Autodesk Fusion 360 part; units mm, degrees
(part 4 of 7)
  line L862 (59.3577, -70.4134) -> (59.3622, -70.4873)
  line L863 (59.3622, -70.4873) -> (59.3692, -70.5616)
  line L864 (59.3692, -70.5616) -> (59.3786, -70.6363)
  line L865 (59.3786, -70.6363) -> (59.3901, -70.7113)
  line L866 (59.3901, -70.7113) -> (59.4036, -70.7865)
  line L867 (59.4036, -70.7865) -> (59.4191, -70.8621)
  line L868 (59.4191, -70.8621) -> (59.4365, -70.9378)
  line L869 (59.4365, -70.9378) -> (59.4556, -71.0137)
  line L870 (59.4556, -71.0137) -> (59.4765, -71.0898)
  line L871 (59.4765, -71.0898) -> (59.6154, -71.1105)
  line L872 (59.6154, -71.1105) -> (59.7546, -71.1291)
  line L873 (59.7546, -71.1291) -> (59.8941, -71.1456)
  line L874 (59.8941, -71.1456) -> (59.9342, -71.0776)
  line L875 (59.9342, -71.0776) -> (59.9726, -71.0093)
  line L876 (59.9726, -71.0093) -> (60.0092, -70.9408)
  line L877 (60.0092, -70.9408) -> (60.044, -70.872)
  line L878 (60.044, -70.872) -> (60.0768, -70.8029)
  line L879 (60.0768, -70.8029) -> (60.1076, -70.7336)
  line L880 (60.1076, -70.7336) -> (60.1362, -70.6639)
  line L881 (60.1362, -70.6639) -> (60.1624, -70.5941)
  line L882 (60.1624, -70.5941) -> (60.1862, -70.524)
  line L883 (60.1862, -70.524) -> (60.207, -70.4536)
  line L884 (60.207, -70.4536) -> (60.2243, -70.3828)
  line L885 (60.2243, -70.3828) -> (60.2364, -70.3117)
  line L886 (60.2364, -70.3117) -> (60.2724, -69.8659)
  line L887 (60.2724, -69.8659) -> (60.483, -69.8801)
  line L888 (60.483, -69.8801) -> (60.694, -69.8888)
  line L889 (60.694, -69.8888) -> (60.9051, -69.8919)
  line L890 (60.9051, -69.8919) -> (61.1162, -69.8895)
  line L891 (61.1162, -69.8895) -> (61.1273, -70.3366)
  line L892 (61.1273, -70.3366) -> (61.1353, -70.4083)
  line L893 (61.1353, -70.4083) -> (61.1487, -70.4799)
  line L894 (61.1487, -70.4799) -> (61.1655, -70.5513)
  line L895 (61.1655, -70.5513) -> (61.1853, -70.6227)
  line L896 (61.1853, -70.6227) -> (61.2076, -70.6939)
  line L897 (61.2076, -70.6939) -> (61.2323, -70.765)
  line L898 (61.2323, -70.765) -> (61.2592, -70.8359)
  line L899 (61.2592, -70.8359) -> (61.2881, -70.9067)
  line L900 (61.2881, -70.9067) -> (61.3189, -70.9774)
  line L901 (61.3189, -70.9774) -> (61.3516, -71.0479)
  line L902 (61.3516, -71.0479) -> (61.3862, -71.1182)
  line L903 (61.3862, -71.1182) -> (61.4225, -71.1882)
  line L904 (61.4225, -71.1882) -> (61.5626, -71.1796)
  line L905 (61.5626, -71.1796) -> (61.7026, -71.1688)
  line L906 (61.7026, -71.1688) -> (61.8425, -71.1559)
  line L907 (61.8425, -71.1559) -> (61.8676, -71.0811)
  line L908 (61.8676, -71.0811) -> (61.891, -71.0064)
  line L909 (61.891, -71.0064) -> (61.9125, -70.9317)
  line L910 (61.9125, -70.9317) -> (61.9322, -70.8572)
  line L911 (61.9322, -70.8572) -> (61.9499, -70.7828)
  line L912 (61.9499, -70.7828) -> (61.9656, -70.7086)
  line L913 (61.9656, -70.7086) -> (61.9791, -70.6345)
  line L914 (61.9791, -70.6345) -> (61.9903, -70.5607)
  line L915 (61.9903, -70.5607) -> (61.9989, -70.4872)
  line L916 (61.9989, -70.4872) -> (62.0047, -70.414)
  line L917 (62.0047, -70.414) -> (62.0069, -70.3412)
  line L918 (62.0069, -70.3412) -> (62.0039, -70.2691)
  line L919 (62.0039, -70.2691) -> (61.9464, -69.8256)
  line L920 (61.9464, -69.8256) -> (62.1554, -69.7957)
  line L921 (62.1554, -69.7957) -> (62.3636, -69.7603)
  line L922 (62.3636, -69.7603) -> (62.5707, -69.7195)
  line L923 (62.5707, -69.7195) -> (62.7767, -69.6732)
  line L924 (62.7767, -69.6732) -> (62.8805, -70.1082)
  line L925 (62.8805, -70.1082) -> (62.9033, -70.1767)
  line L926 (62.9033, -70.1767) -> (62.9312, -70.2439)
  line L927 (62.9312, -70.2439) -> (62.9626, -70.3103)
  line L928 (62.9626, -70.3103) -> (62.9968, -70.376)
  line L929 (62.9968, -70.376) -> (63.0334, -70.441)
  line L930 (63.0334, -70.441) -> (63.0723, -70.5054)
  line L931 (63.0723, -70.5054) -> (63.1133, -70.5693)
  line L932 (63.1133, -70.5693) -> (63.1563, -70.6325)
  line L933 (63.1563, -70.6325) -> (63.2012, -70.6952)
  line L934 (63.2012, -70.6952) -> (63.2479, -70.7573)
  line L935 (63.2479, -70.7573) -> (63.2963, -70.8189)
  line L936 (63.2963, -70.8189) -> (63.3463, -70.8799)
  line L937 (63.3463, -70.8799) -> (63.4816, -70.8423)
  line L938 (63.4816, -70.8423) -> (63.6163, -70.8027)
  line L939 (63.6163, -70.8027) -> (63.7504, -70.761)
  line L940 (63.7504, -70.761) -> (63.7595, -70.6826)
  line L941 (63.7595, -70.6826) -> (63.7668, -70.6046)
  line L942 (63.7668, -70.6046) -> (63.7723, -70.5271)
  line L943 (63.7723, -70.5271) -> (63.7761, -70.4501)
  line L944 (63.7761, -70.4501) -> (63.778, -70.3736)
  line L945 (63.778, -70.3736) -> (63.7779, -70.2978)
  line L946 (63.7779, -70.2978) -> (63.7757, -70.2226)
  line L947 (63.7757, -70.2226) -> (63.7713, -70.148)
  line L948 (63.7713, -70.148) -> (63.7644, -70.0743)
  line L949 (63.7644, -70.0743) -> (63.7548, -70.0015)
  line L950 (63.7548, -70.0015) -> (63.7419, -69.9299)
  line L951 (63.7419, -69.9299) -> (63.7239, -69.86)
  line L952 (63.7239, -69.86) -> (63.5755, -69.4381)
  line L953 (63.5755, -69.4381) -> (63.7738, -69.3654)
  line L954 (63.7738, -69.3654) -> (63.97, -69.2875)
  line L955 (63.97, -69.2875) -> (64.1641, -69.2045)
  line L956 (64.1641, -69.2045) -> (64.356, -69.1164)
  line L957 (64.356, -69.1164) -> (64.548, -69.5204)
  line L958 (64.548, -69.5204) -> (64.5845, -69.5826)
  line L959 (64.5845, -69.5826) -> (64.6258, -69.6425)
  line L960 (64.6258, -69.6425) -> (64.6703, -69.701)
  line L961 (64.6703, -69.701) -> (64.7173, -69.7581)
  line L962 (64.7173, -69.7581) -> (64.7667, -69.8141)
  line L963 (64.7667, -69.8141) -> (64.8182, -69.869)
  line L964 (64.8182, -69.869) -> (64.8716, -69.9229)
  line L965 (64.8716, -69.9229) -> (64.9268, -69.9758)
  line L966 (64.9268, -69.9758) -> (64.9837, -70.0278)
  line L967 (64.9837, -70.0278) -> (65.0422, -70.0789)
  line L968 (65.0422, -70.0789) -> (65.1024, -70.1291)
  line L969 (65.1024, -70.1291) -> (65.164, -70.1783)
  line L970 (65.164, -70.1783) -> (65.2886, -70.1134)
  line L971 (65.2886, -70.1134) -> (65.4121, -70.0466)
  line L972 (65.4121, -70.0466) -> (65.5346, -69.978)
  line L973 (65.5346, -69.978) -> (65.5271, -69.8994)
  line L974 (65.5271, -69.8994) -> (65.5181, -69.8216)
  line L975 (65.5181, -69.8216) -> (65.5074, -69.7447)
  line L976 (65.5074, -69.7447) -> (65.4951, -69.6686)
  line L977 (65.4951, -69.6686) -> (65.481, -69.5934)
  line L978 (65.481, -69.5934) -> (65.4651, -69.5192)
  line L979 (65.4651, -69.5192) -> (65.4473, -69.4461)
  line L980 (65.4473, -69.4461) -> (65.4275, -69.3741)
  line L981 (65.4275, -69.3741) -> (65.4055, -69.3034)
  line L982 (65.4055, -69.3034) -> (65.381, -69.2342)
  line L983 (65.381, -69.2342) -> (65.3534, -69.1668)
  line L984 (65.3534, -69.1668) -> (65.3213, -69.1022)
  line L985 (65.3213, -69.1022) -> (65.0885, -68.7204)
  line L986 (65.0885, -68.7204) -> (65.2673, -68.6081)
  line L987 (65.2673, -68.6081) -> (65.443, -68.4911)
  line L988 (65.443, -68.4911) -> (65.6156, -68.3695)
  line L989 (65.6156, -68.3695) -> (65.785, -68.2435)
extrude "Extrude1''" add sketch "Sketch1 (3)" along normal blind 1.8 separate body makes body 4 in component "CT idler 2"
ref_plane "WorkPlane2" through (0, 0, 40.8) normal (0, 0, 1) x (1, 0, 0) in component "CT idler 2"
sketch "Sketch2 (2)" plane through (0, 0, 40.8) normal (0, 0, 1) x (1, 0, 0) in component "CT idler 2"
  line L0 (63.9904, -61.5562) -> (64.2817, -61.5253)
  line L1 (64.2817, -61.5253) -> (64.3597, -61.5053)
  line L2 (64.3597, -61.5053) -> (64.4366, -61.4752)
  line L3 (64.4366, -61.4752) -> (64.5125, -61.4382)
  line L4 (64.5125, -61.4382) -> (64.5874, -61.3953)
  line L5 (64.5874, -61.3953) -> (64.6613, -61.3471)
  line L6 (64.6613, -61.3471) -> (64.734, -61.2939)
  line L7 (64.734, -61.2939) -> (64.8056, -61.2361)
  line L8 (64.8056, -61.2361) -> (64.8757, -61.1738)
  line L9 (64.8757, -61.1738) -> (64.9445, -61.1072)
  line L10 (64.9445, -61.1072) -> (65.0117, -61.0364)
  line L11 (65.0117, -61.0364) -> (65.0773, -60.9615)
  line L12 (65.0773, -60.9615) -> (65.141, -60.8827)
  line L13 (65.141, -60.8827) -> (65.1206, -60.7999)
  line L14 (65.1206, -60.7999) -> (65.0985, -60.7175)
  line L15 (65.0985, -60.7175) -> (65.0748, -60.6356)
  line L16 (65.0748, -60.6356) -> (64.9802, -60.5992)
  line L17 (64.9802, -60.5992) -> (64.886, -60.5672)
  line L18 (64.886, -60.5672) -> (64.7924, -60.5395)
  line L19 (64.7924, -60.5395) -> (64.6995, -60.5161)
  line L20 (64.6995, -60.5161) -> (64.6076, -60.4973)
  line L21 (64.6076, -60.4973) -> (64.5167, -60.4829)
  line L22 (64.5167, -60.4829) -> (64.4272, -60.4733)
  line L23 (64.4272, -60.4733) -> (64.3391, -60.4685)
  line L24 (64.3391, -60.4685) -> (64.2528, -60.4688)
  line L25 (64.2528, -60.4688) -> (64.1685, -60.4747)
  line L26 (64.1685, -60.4747) -> (64.0869, -60.4871)
  line L27 (64.0869, -60.4871) -> (64.0093, -60.5088)
  line L28 (64.0093, -60.5088) -> (63.7416, -60.6277)
  line L29 (63.7416, -60.6277) -> (63.6715, -60.4803)
  line L30 (63.6715, -60.4803) -> (63.5936, -60.3369)
  line L31 (63.5936, -60.3369) -> (63.5084, -60.1978)
  line L32 (63.5084, -60.1978) -> (63.4159, -60.0634)
  line L33 (63.4159, -60.0634) -> (63.6527, -59.8911)
  line L34 (63.6527, -59.8911) -> (63.7102, -59.8347)
  line L35 (63.7102, -59.8347) -> (63.7618, -59.7702)
  line L36 (63.7618, -59.7702) -> (63.809, -59.7002)
  line L37 (63.809, -59.7002) -> (63.8525, -59.6256)
  line L38 (63.8525, -59.6256) -> (63.8923, -59.5469)
  line L39 (63.8923, -59.5469) -> (63.9287, -59.4645)
  line L40 (63.9287, -59.4645) -> (63.9618, -59.3787)
  line L41 (63.9618, -59.3787) -> (63.9914, -59.2896)
  line L42 (63.9914, -59.2896) -> (64.0176, -59.1975)
  line L43 (64.0176, -59.1975) -> (64.0404, -59.1026)
  line L44 (64.0404, -59.1026) -> (64.0598, -59.005)
  line L45 (64.0598, -59.005) -> (64.0756, -58.9049)
  line L46 (64.0756, -58.9049) -> (64.0165, -58.8434)
  line L47 (64.0165, -58.8434) -> (63.9562, -58.7831)
  line L48 (63.9562, -58.7831) -> (63.8947, -58.724)
  line L49 (63.8947, -58.724) -> (63.7945, -58.7398)
  line L50 (63.7945, -58.7398) -> (63.6969, -58.7591)
  line L51 (63.6969, -58.7591) -> (63.602, -58.7819)
  line L52 (63.602, -58.7819) -> (63.51, -58.8082)
  line L53 (63.51, -58.8082) -> (63.4209, -58.8378)
  line L54 (63.4209, -58.8378) -> (63.3351, -58.8708)
  line L55 (63.3351, -58.8708) -> (63.2526, -58.9072)
  line L56 (63.2526, -58.9072) -> (63.174, -58.9471)
  line L57 (63.174, -58.9471) -> (63.0994, -58.9905)
  line L58 (63.0994, -58.9905) -> (63.0294, -59.0378)
  line L59 (63.0294, -59.0378) -> (62.9649, -59.0893)
  line L60 (62.9649, -59.0893) -> (62.9085, -59.1469)
  line L61 (62.9085, -59.1469) -> (62.7361, -59.3837)
  line L62 (62.7361, -59.3837) -> (62.6017, -59.2912)
  line L63 (62.6017, -59.2912) -> (62.4626, -59.2059)
  line L64 (62.4626, -59.2059) -> (62.3192, -59.1281)
  line L65 (62.3192, -59.1281) -> (62.1719, -59.0579)
  line L66 (62.1719, -59.0579) -> (62.2908, -58.7903)
  line L67 (62.2908, -58.7903) -> (62.3125, -58.7126)
  line L68 (62.3125, -58.7126) -> (62.3249, -58.631)
  line L69 (62.3249, -58.631) -> (62.3308, -58.5468)
  line L70 (62.3308, -58.5468) -> (62.3311, -58.4605)
  line L71 (62.3311, -58.4605) -> (62.3263, -58.3724)
  line L72 (62.3263, -58.3724) -> (62.3166, -58.2828)
  line L73 (62.3166, -58.2828) -> (62.3023, -58.192)
  line L74 (62.3023, -58.192) -> (62.2834, -58.1)
  line L75 (62.2834, -58.1) -> (62.2601, -58.0072)
  line L76 (62.2601, -58.0072) -> (62.2324, -57.9136)
  line L77 (62.2324, -57.9136) -> (62.2003, -57.8194)
  line L78 (62.2003, -57.8194) -> (62.164, -57.7247)
  line L79 (62.164, -57.7247) -> (62.082, -57.7011)
  line L80 (62.082, -57.7011) -> (61.9996, -57.679)
  line L81 (61.9996, -57.679) -> (61.9168, -57.6585)
  line L82 (61.9168, -57.6585) -> (61.838, -57.7223)
  line L83 (61.838, -57.7223) -> (61.7632, -57.7879)
  line L84 (61.7632, -57.7879) -> (61.6924, -57.8551)
  line L85 (61.6924, -57.8551) -> (61.6258, -57.9238)
  line L86 (61.6258, -57.9238) -> (61.5635, -57.994)
  line L87 (61.5635, -57.994) -> (61.5056, -58.0655)
  line L88 (61.5056, -58.0655) -> (61.4525, -58.1383)
  line L89 (61.4525, -58.1383) -> (61.4043, -58.2121)
  line L90 (61.4043, -58.2121) -> (61.3614, -58.287)
  line L91 (61.3614, -58.287) -> (61.3244, -58.3629)
  line L92 (61.3244, -58.3629) -> (61.2943, -58.4398)
  line L93 (61.2943, -58.4398) -> (61.2743, -58.5179)
  line L94 (61.2743, -58.5179) -> (61.2434, -58.8091)
  line L95 (61.2434, -58.8091) -> (61.0807, -58.7962)
  line L96 (61.0807, -58.7962) -> (60.9176, -58.7919)
  line L97 (60.9176, -58.7919) -> (60.7545, -58.7962)
  line L98 (60.7545, -58.7962) -> (60.5919, -58.8091)
  line L99 (60.5919, -58.8091) -> (60.561, -58.5179)
  line L100 (60.561, -58.5179) -> (60.541, -58.4398)
  line L101 (60.541, -58.4398) -> (60.5109, -58.3629)
  line L102 (60.5109, -58.3629) -> (60.4739, -58.287)
  line L103 (60.4739, -58.287) -> (60.431, -58.2121)
  line L104 (60.431, -58.2121) -> (60.3828, -58.1383)
  line L105 (60.3828, -58.1383) -> (60.3296, -58.0655)
  line L106 (60.3296, -58.0655) -> (60.2718, -57.994)
  line L107 (60.2718, -57.994) -> (60.2095, -57.9238)
  line L108 (60.2095, -57.9238) -> (60.1429, -57.8551)
  line L109 (60.1429, -57.8551) -> (60.0721, -57.7879)
  line L110 (60.0721, -57.7879) -> (59.9972, -57.7223)
  line L111 (59.9972, -57.7223) -> (59.9184, -57.6585)
  line L112 (59.9184, -57.6585) -> (59.8356, -57.679)
  line L113 (59.8356, -57.679) -> (59.7532, -57.7011)
  line L114 (59.7532, -57.7011) -> (59.6713, -57.7247)
  line L115 (59.6713, -57.7247) -> (59.6349, -57.8194)
  line L116 (59.6349, -57.8194) -> (59.6029, -57.9136)
  line L117 (59.6029, -57.9136) -> (59.5752, -58.0072)
  line L118 (59.5752, -58.0072) -> (59.5518, -58.1)
  line L119 (59.5518, -58.1) -> (59.533, -58.192)
  line L120 (59.533, -58.192) -> (59.5186, -58.2828)
  line L121 (59.5186, -58.2828) -> (59.509, -58.3724)
  line L122 (59.509, -58.3724) -> (59.5042, -58.4605)
  line L123 (59.5042, -58.4605) -> (59.5045, -58.5468)
  line L124 (59.5045, -58.5468) -> (59.5104, -58.631)
  line L125 (59.5104, -58.631) -> (59.5228, -58.7126)
  line L126 (59.5228, -58.7126) -> (59.5445, -58.7903)
  line L127 (59.5445, -58.7903) -> (59.6633, -59.0579)
  line L128 (59.6633, -59.0579) -> (59.516, -59.1281)
  line L129 (59.516, -59.1281) -> (59.3726, -59.2059)
  line L130 (59.3726, -59.2059) -> (59.2335, -59.2912)
  line L131 (59.2335, -59.2912) -> (59.0991, -59.3837)
  line L132 (59.0991, -59.3837) -> (58.9267, -59.1469)
  line L133 (58.9267, -59.1469) -> (58.8704, -59.0893)
  line L134 (58.8704, -59.0893) -> (58.8059, -59.0378)
  line L135 (58.8059, -59.0378) -> (58.7359, -58.9905)
  line L136 (58.7359, -58.9905) -> (58.6613, -58.9471)
  line L137 (58.6613, -58.9471) -> (58.5826, -58.9072)
  line L138 (58.5826, -58.9072) -> (58.5002, -58.8708)
  line L139 (58.5002, -58.8708) -> (58.4144, -58.8378)
  line L140 (58.4144, -58.8378) -> (58.3253, -58.8082)
  line L141 (58.3253, -58.8082) -> (58.2332, -58.7819)
  line L142 (58.2332, -58.7819) -> (58.1383, -58.7591)
  line L143 (58.1383, -58.7591) -> (58.0407, -58.7398)
  line L144 (58.0407, -58.7398) -> (57.9406, -58.724)
  line L145 (57.9406, -58.724) -> (57.8791, -58.7831)
  line L146 (57.8791, -58.7831) -> (57.8188, -58.8434)
  line L147 (57.8188, -58.8434) -> (57.7597, -58.9049)
  line L148 (57.7597, -58.9049) -> (57.7755, -59.005)
  line L149 (57.7755, -59.005) -> (57.7948, -59.1026)
  line L150 (57.7948, -59.1026) -> (57.8176, -59.1975)
  line L151 (57.8176, -59.1975) -> (57.8439, -59.2896)
  line L152 (57.8439, -59.2896) -> (57.8735, -59.3787)
  line L153 (57.8735, -59.3787) -> (57.9065, -59.4645)
  line L154 (57.9065, -59.4645) -> (57.9429, -59.5469)
  line L155 (57.9429, -59.5469) -> (57.9828, -59.6256)
  line L156 (57.9828, -59.6256) -> (58.0262, -59.7002)
  line L157 (58.0262, -59.7002) -> (58.0735, -59.7702)
  line L158 (58.0735, -59.7702) -> (58.125, -59.8347)
  line L159 (58.125, -59.8347) -> (58.1826, -59.8911)
  line L160 (58.1826, -59.8911) -> (58.4194, -60.0634)
  line L161 (58.4194, -60.0634) -> (58.3269, -60.1978)
  line L162 (58.3269, -60.1978) -> (58.2416, -60.3369)
  line L163 (58.2416, -60.3369) -> (58.1638, -60.4803)
  line L164 (58.1638, -60.4803) -> (58.0936, -60.6277)
  line L165 (58.0936, -60.6277) -> (57.826, -60.5088)
  line L166 (57.826, -60.5088) -> (57.7483, -60.4871)
  line L167 (57.7483, -60.4871) -> (57.6667, -60.4747)
  line L168 (57.6667, -60.4747) -> (57.5825, -60.4688)
  line L169 (57.5825, -60.4688) -> (57.4962, -60.4685)
  line L170 (57.4962, -60.4685) -> (57.4081, -60.4733)
  line L171 (57.4081, -60.4733) -> (57.3185, -60.4829)
  line L172 (57.3185, -60.4829) -> (57.2277, -60.4973)
  line L173 (57.2277, -60.4973) -> (57.1357, -60.5161)
  line L174 (57.1357, -60.5161) -> (57.0429, -60.5395)
  line L175 (57.0429, -60.5395) -> (56.9493, -60.5672)
  line L176 (56.9493, -60.5672) -> (56.8551, -60.5992)
  line L177 (56.8551, -60.5992) -> (56.7604, -60.6356)
  line L178 (56.7604, -60.6356) -> (56.7367, -60.7175)
  line L179 (56.7367, -60.7175) -> (56.7147, -60.7999)
  line L180 (56.7147, -60.7999) -> (56.6942, -60.8827)
  line L181 (56.6942, -60.8827) -> (56.758, -60.9615)
  line L182 (56.758, -60.9615) -> (56.8235, -61.0364)
  line L183 (56.8235, -61.0364) -> (56.8908, -61.1072)
  line L184 (56.8908, -61.1072) -> (56.9595, -61.1738)
  line L185 (56.9595, -61.1738) -> (57.0297, -61.2361)
  line L186 (57.0297, -61.2361) -> (57.1012, -61.2939)
  line L187 (57.1012, -61.2939) -> (57.1739, -61.3471)
  line L188 (57.1739, -61.3471) -> (57.2478, -61.3953)
  line L189 (57.2478, -61.3953) -> (57.3227, -61.4382)
  line L190 (57.3227, -61.4382) -> (57.3986, -61.4752)
  line L191 (57.3986, -61.4752) -> (57.4755, -61.5053)
  line L192 (57.4755, -61.5053) -> (57.5536, -61.5253)
  line L193 (57.5536, -61.5253) -> (57.8448, -61.5562)
  line L194 (57.8448, -61.5562) -> (57.8319, -61.7188)
  line L195 (57.8319, -61.7188) -> (57.8276, -61.8819)
  line L196 (57.8276, -61.8819) -> (57.8319, -62.045)
  line L197 (57.8319, -62.045) -> (57.8448, -62.2077)
  line L198 (57.8448, -62.2077) -> (57.5536, -62.2386)
  line L199 (57.5536, -62.2386) -> (57.4755, -62.2586)
  line L200 (57.4755, -62.2586) -> (57.3986, -62.2887)
  line L201 (57.3986, -62.2887) -> (57.3227, -62.3257)
  line L202 (57.3227, -62.3257) -> (57.2478, -62.3686)
  line L203 (57.2478, -62.3686) -> (57.1739, -62.4168)
  line L204 (57.1739, -62.4168) -> (57.1012, -62.4699)
  line L205 (57.1012, -62.4699) -> (57.0297, -62.5278)
  line L206 (57.0297, -62.5278) -> (56.9595, -62.5901)
  line L207 (56.9595, -62.5901) -> (56.8908, -62.6567)
  line L208 (56.8908, -62.6567) -> (56.8235, -62.7275)
  line L209 (56.8235, -62.7275) -> (56.758, -62.8023)
  line L210 (56.758, -62.8023) -> (56.6942, -62.8811)
  line L211 (56.6942, -62.8811) -> (56.7147, -62.964)
  line L212 (56.7147, -62.964) -> (56.7367, -63.0463)
  line L213 (56.7367, -63.0463) -> (56.7604, -63.1283)
  line L214 (56.7604, -63.1283) -> (56.8551, -63.1646)
  line L215 (56.8551, -63.1646) -> (56.9493, -63.1967)
  line L216 (56.9493, -63.1967) -> (57.0429, -63.2244)
  line L217 (57.0429, -63.2244) -> (57.1357, -63.2477)
  line L218 (57.1357, -63.2477) -> (57.2277, -63.2666)
  line L219 (57.2277, -63.2666) -> (57.3185, -63.2809)
  line L220 (57.3185, -63.2809) -> (57.4081, -63.2906)
  line L221 (57.4081, -63.2906) -> (57.4962, -63.2954)
  line L222 (57.4962, -63.2954) -> (57.5825, -63.2951)
  line L223 (57.5825, -63.2951) -> (57.6667, -63.2892)
  line L224 (57.6667, -63.2892) -> (57.7483, -63.2768)
  line L225 (57.7483, -63.2768) -> (57.826, -63.2551)
  line L226 (57.826, -63.2551) -> (58.0936, -63.1362)
  line L227 (58.0936, -63.1362) -> (58.1638, -63.2835)
  line L228 (58.1638, -63.2835) -> (58.2416, -63.4269)
  line L229 (58.2416, -63.4269) -> (58.3269, -63.566)
  line L230 (58.3269, -63.566) -> (58.4194, -63.7004)
  line L231 (58.4194, -63.7004) -> (58.1826, -63.8728)
  line L232 (58.1826, -63.8728) -> (58.125, -63.9292)
  line L233 (58.125, -63.9292) -> (58.0735, -63.9937)
  line L234 (58.0735, -63.9937) -> (58.0262, -64.0637)
  line L235 (58.0262, -64.0637) -> (57.9828, -64.1383)
  line L236 (57.9828, -64.1383) -> (57.9429, -64.217)
  line L237 (57.9429, -64.217) -> (57.9065, -64.2994)
  line L238 (57.9065, -64.2994) -> (57.8735, -64.3852)
  line L239 (57.8735, -64.3852) -> (57.8439, -64.4743)
  line L240 (57.8439, -64.4743) -> (57.8176, -64.5663)
  line L241 (57.8176, -64.5663) -> (57.7948, -64.6612)
  line L242 (57.7948, -64.6612) -> (57.7755, -64.7588)
  line L243 (57.7755, -64.7588) -> (57.7597, -64.859)
  line L244 (57.7597, -64.859) -> (57.8188, -64.9205)
  line L245 (57.8188, -64.9205) -> (57.8791, -64.9808)
  line L246 (57.8791, -64.9808) -> (57.9406, -65.0399)
  line L247 (57.9406, -65.0399) -> (58.0407, -65.0241)
  line L248 (58.0407, -65.0241) -> (58.1383, -65.0047)
  line L249 (58.1383, -65.0047) -> (58.2332, -64.9819)
  line L250 (58.2332, -64.9819) -> (58.3253, -64.9557)
  line L251 (58.3253, -64.9557) -> (58.4144, -64.9261)
  line L252 (58.4144, -64.9261) -> (58.5002, -64.893)
  line L253 (58.5002, -64.893) -> (58.5826, -64.8566)
  line L254 (58.5826, -64.8566) -> (58.6613, -64.8168)
  line L255 (58.6613, -64.8168) -> (58.7359, -64.7733)
  line L256 (58.7359, -64.7733) -> (58.8059, -64.7261)
  line L257 (58.8059, -64.7261) -> (58.8704, -64.6745)
  line L258 (58.8704, -64.6745) -> (58.9267, -64.617)
  line L259 (58.9267, -64.617) -> (59.0991, -64.3802)
  line L260 (59.0991, -64.3802) -> (59.2335, -64.4727)
  line L261 (59.2335, -64.4727) -> (59.3726, -64.5579)
  line L262 (59.3726, -64.5579) -> (59.516, -64.6358)
  line L263 (59.516, -64.6358) -> (59.6633, -64.7059)
  line L264 (59.6633, -64.7059) -> (59.5445, -64.9736)
  line L265 (59.5445, -64.9736) -> (59.5228, -65.0512)
  line L266 (59.5228, -65.0512) -> (59.5104, -65.1328)
  line L267 (59.5104, -65.1328) -> (59.5045, -65.2171)
  line L268 (59.5045, -65.2171) -> (59.5042, -65.3034)
  line L269 (59.5042, -65.3034) -> (59.509, -65.3915)
  line L270 (59.509, -65.3915) -> (59.5186, -65.481)
  line L271 (59.5186, -65.481) -> (59.533, -65.5719)
  line L272 (59.533, -65.5719) -> (59.5518, -65.6638)
  line L273 (59.5518, -65.6638) -> (59.5752, -65.7567)
  line L274 (59.5752, -65.7567) -> (59.6029, -65.8503)
  line L275 (59.6029, -65.8503) -> (59.6349, -65.9445)
  line L276 (59.6349, -65.9445) -> (59.6713, -66.0391)
  line L277 (59.6713, -66.0391) -> (59.7532, -66.0628)
  line L278 (59.7532, -66.0628) -> (59.8356, -66.0849)
  line L279 (59.8356, -66.0849) -> (59.9184, -66.1053)
  line L280 (59.9184, -66.1053) -> (59.9972, -66.0416)
  line L281 (59.9972, -66.0416) -> (60.0721, -65.976)
  line L282 (60.0721, -65.976) -> (60.1429, -65.9088)
  line L283 (60.1429, -65.9088) -> (60.2095, -65.84)
  line L284 (60.2095, -65.84) -> (60.2718, -65.7699)
  line L285 (60.2718, -65.7699) -> (60.3296, -65.6983)
  line L286 (60.3296, -65.6983) -> (60.3828, -65.6256)
  line L287 (60.3828, -65.6256) -> (60.431, -65.5517)
  line L288 (60.431, -65.5517) -> (60.4739, -65.4768)
  line L289 (60.4739, -65.4768) -> (60.5109, -65.4009)
  line L290 (60.5109, -65.4009) -> (60.541, -65.324)
  line L291 (60.541, -65.324) -> (60.561, -65.246)
  line L292 (60.561, -65.246) -> (60.5919, -64.9547)
  line L293 (60.5919, -64.9547) -> (60.7545, -64.9676)
  line L294 (60.7545, -64.9676) -> (60.9176, -64.9719)
  line L295 (60.9176, -64.9719) -> (61.0807, -64.9676)
  line L296 (61.0807, -64.9676) -> (61.2434, -64.9547)
  line L297 (61.2434, -64.9547) -> (61.2743, -65.246)
  line L298 (61.2743, -65.246) -> (61.2943, -65.324)
  line L299 (61.2943, -65.324) -> (61.3244, -65.4009)
  line L300 (61.3244, -65.4009) -> (61.3614, -65.4768)
  line L301 (61.3614, -65.4768) -> (61.4043, -65.5517)
  line L302 (61.4043, -65.5517) -> (61.4525, -65.6256)
  line L303 (61.4525, -65.6256) -> (61.5056, -65.6983)
  line L304 (61.5056, -65.6983) -> (61.5635, -65.7699)
  line L305 (61.5635, -65.7699) -> (61.6258, -65.84)
  line L306 (61.6258, -65.84) -> (61.6924, -65.9088)
  line L307 (61.6924, -65.9088) -> (61.7632, -65.976)
  line L308 (61.7632, -65.976) -> (61.838, -66.0416)
  line L309 (61.838, -66.0416) -> (61.9168, -66.1053)
  line L310 (61.9168, -66.1053) -> (61.9996, -66.0849)
  line L311 (61.9996, -66.0849) -> (62.082, -66.0628)
  line L312 (62.082, -66.0628) -> (62.164, -66.0391)
  line L313 (62.164, -66.0391) -> (62.2003, -65.9445)
  line L314 (62.2003, -65.9445) -> (62.2324, -65.8503)
  line L315 (62.2324, -65.8503) -> (62.2601, -65.7567)
  line L316 (62.2601, -65.7567) -> (62.2834, -65.6638)
  line L317 (62.2834, -65.6638) -> (62.3023, -65.5719)
  line L318 (62.3023, -65.5719) -> (62.3166, -65.481)
  line L319 (62.3166, -65.481) -> (62.3263, -65.3915)
  line L320 (62.3263, -65.3915) -> (62.3311, -65.3034)
  line L321 (62.3311, -65.3034) -> (62.3308, -65.2171)
  line L322 (62.3308, -65.2171) -> (62.3249, -65.1328)
  line L323 (62.3249, -65.1328) -> (62.3125, -65.0512)
  line L324 (62.3125, -65.0512) -> (62.2908, -64.9736)
  line L325 (62.2908, -64.9736) -> (62.1719, -64.7059)
  line L326 (62.1719, -64.7059) -> (62.3192, -64.6358)
  line L327 (62.3192, -64.6358) -> (62.4626, -64.5579)
  line L328 (62.4626, -64.5579) -> (62.6017, -64.4727)
  line L329 (62.6017, -64.4727) -> (62.7361, -64.3802)
  line L330 (62.7361, -64.3802) -> (62.9085, -64.617)
  line L331 (62.9085, -64.617) -> (62.9649, -64.6745)
  line L332 (62.9649, -64.6745) -> (63.0294, -64.7261)
  line L333 (63.0294, -64.7261) -> (63.0994, -64.7733)
  line L334 (63.0994, -64.7733) -> (63.174, -64.8168)
  line L335 (63.174, -64.8168) -> (63.2526, -64.8566)
  line L336 (63.2526, -64.8566) -> (63.3351, -64.893)
  line L337 (63.3351, -64.893) -> (63.4209, -64.9261)
  line L338 (63.4209, -64.9261) -> (63.51, -64.9557)
  line L339 (63.51, -64.9557) -> (63.602, -64.9819)
  line L340 (63.602, -64.9819) -> (63.6969, -65.0047)
  line L341 (63.6969, -65.0047) -> (63.7945, -65.0241)
  line L342 (63.7945, -65.0241) -> (63.8947, -65.0399)
  line L343 (63.8947, -65.0399) -> (63.9562, -64.9808)
  line L344 (63.9562, -64.9808) -> (64.0165, -64.9205)
  line L345 (64.0165, -64.9205) -> (64.0756, -64.859)
  line L346 (64.0756, -64.859) -> (64.0598, -64.7588)
  line L347 (64.0598, -64.7588) -> (64.0404, -64.6612)
  line L348 (64.0404, -64.6612) -> (64.0176, -64.5663)
  line L349 (64.0176, -64.5663) -> (63.9914, -64.4743)
  line L350 (63.9914, -64.4743) -> (63.9618, -64.3852)
  line L351 (63.9618, -64.3852) -> (63.9287, -64.2994)
  line L352 (63.9287, -64.2994) -> (63.8923, -64.217)
  line L353 (63.8923, -64.217) -> (63.8525, -64.1383)
  line L354 (63.8525, -64.1383) -> (63.809, -64.0637)
  line L355 (63.809, -64.0637) -> (63.7618, -63.9937)
  line L356 (63.7618, -63.9937) -> (63.7102, -63.9292)
  line L357 (63.7102, -63.9292) -> (63.6527, -63.8728)
  line L358 (63.6527, -63.8728) -> (63.4159, -63.7004)
  line L359 (63.4159, -63.7004) -> (63.5084, -63.566)
  line L360 (63.5084, -63.566) -> (63.5936, -63.4269)
  line L361 (63.5936, -63.4269) -> (63.6715, -63.2835)
  line L362 (63.6715, -63.2835) -> (63.7416, -63.1362)
  line L363 (63.7416, -63.1362) -> (64.0093, -63.2551)
  line L364 (64.0093, -63.2551) -> (64.0869, -63.2768)
  line L365 (64.0869, -63.2768) -> (64.1685, -63.2892)
  line L366 (64.1685, -63.2892) -> (64.2528, -63.2951)
  line L367 (64.2528, -63.2951) -> (64.3391, -63.2954)
  line L368 (64.3391, -63.2954) -> (64.4272, -63.2906)
  line L369 (64.4272, -63.2906) -> (64.5167, -63.2809)
  line L370 (64.5167, -63.2809) -> (64.6076, -63.2666)
  line L371 (64.6076, -63.2666) -> (64.6995, -63.2477)
  line L372 (64.6995, -63.2477) -> (64.7924, -63.2244)
  line L373 (64.7924, -63.2244) -> (64.886, -63.1967)
  line L374 (64.886, -63.1967) -> (64.9802, -63.1646)
  line L375 (64.9802, -63.1646) -> (65.0748, -63.1283)
  line L376 (65.0748, -63.1283) -> (65.0985, -63.0463)
  line L377 (65.0985, -63.0463) -> (65.1206, -62.964)
  line L378 (65.1206, -62.964) -> (65.141, -62.8811)
  line L379 (65.141, -62.8811) -> (65.0773, -62.8023)
  line L380 (65.0773, -62.8023) -> (65.0117, -62.7275)
  line L381 (65.0117, -62.7275) -> (64.9445, -62.6567)
  line L382 (64.9445, -62.6567) -> (64.8757, -62.5901)
  line L383 (64.8757, -62.5901) -> (64.8056, -62.5278)
  line L384 (64.8056, -62.5278) -> (64.734, -62.4699)
  line L385 (64.734, -62.4699) -> (64.6613, -62.4168)
  line L386 (64.6613, -62.4168) -> (64.5874, -62.3686)
  line L387 (64.5874, -62.3686) -> (64.5125, -62.3257)
  line L388 (64.5125, -62.3257) -> (64.4366, -62.2887)
  line L389 (64.4366, -62.2887) -> (64.3597, -62.2586)
  line L390 (64.3597, -62.2586) -> (64.2817, -62.2386)
  line L391 (64.2817, -62.2386) -> (63.9904, -62.2077)
  line L392 (63.9904, -62.2077) -> (64.0033, -62.045)
  line L393 (64.0033, -62.045) -> (64.0076, -61.8819)
  line L394 (64.0076, -61.8819) -> (64.0033, -61.7188)
  line L395 (64.0033, -61.7188) -> (63.9904, -61.5562)
extrude "Extrude2'" add sketch "Sketch2 (2)" along normal blind 2.2 separate body makes body 5 in component "CT idler 2"
combine "Combine1'" operation add target body 4 tool bodies 5 in component "CT idler 2"
ref_plane "WorkPlane3" through (0, 0, 39) normal (0, 0, 1) x (1, 0, 0) in component "CT idler 2"
sketch "Sketch3 (2)" plane through (0, 0, 39) normal (0, 0, 1) x (1, 0, 0) in component "CT idler 2"
  circle A0 centre (60.9176, -61.8819) radius 1.7
extrude "Extrude3'" cut sketch "Sketch3 (2)" along normal blind 4 bodies 4 in component "CT idler 2"
ref_plane "WorkPlane1" through (0, 0, 41.2) normal (0, 0, 1) x (1, 0, 0) in component "CT idler 3"
sketch "Sketch1 (4)" plane through (0, 0, 41.2) normal (0, 0, 1) x (1, 0, 0) in component "CT idler 3"
  line L0 (65.8918, -57.7776) -> (65.959, -58.2198)
  line L1 (65.959, -58.2198) -> (65.9761, -58.2899)
  line L2 (65.9761, -58.2899) -> (65.9983, -58.3592)
  line L3 (65.9983, -58.3592) -> (66.024, -58.428)
  line L4 (66.024, -58.428) -> (66.0526, -58.4963)
  line L5 (66.0526, -58.4963) -> (66.0838, -58.5641)
  line L6 (66.0838, -58.5641) -> (66.1172, -58.6316)
  line L7 (66.1172, -58.6316) -> (66.1528, -58.6986)
  line L8 (66.1528, -58.6986) -> (66.1903, -58.7652)
  line L9 (66.1903, -58.7652) -> (66.2298, -58.8314)
  line L10 (66.2298, -58.8314) -> (66.2712, -58.8972)
  line L11 (66.2712, -58.8972) -> (66.3143, -58.9626)
  line L12 (66.3143, -58.9626) -> (66.3591, -59.0275)
  line L13 (66.3591, -59.0275) -> (66.4971, -59.0013)
  line L14 (66.4971, -59.0013) -> (66.6346, -58.973)
  line L15 (66.6346, -58.973) -> (66.7717, -58.9426)
  line L16 (66.7717, -58.9426) -> (66.7872, -58.8652)
  line L17 (66.7872, -58.8652) -> (66.801, -58.7881)
  line L18 (66.801, -58.7881) -> (66.813, -58.7113)
  line L19 (66.813, -58.7113) -> (66.8231, -58.6349)
  line L20 (66.8231, -58.6349) -> (66.8313, -58.5589)
  line L21 (66.8313, -58.5589) -> (66.8375, -58.4833)
  line L22 (66.8375, -58.4833) -> (66.8416, -58.4081)
  line L23 (66.8416, -58.4081) -> (66.8434, -58.3335)
  line L24 (66.8434, -58.3335) -> (66.8427, -58.2595)
  line L25 (66.8427, -58.2595) -> (66.8392, -58.1861)
  line L26 (66.8392, -58.1861) -> (66.8322, -58.1137)
  line L27 (66.8322, -58.1137) -> (66.8202, -58.0425)
  line L28 (66.8202, -58.0425) -> (66.7074, -57.6097)
  line L29 (66.7074, -57.6097) -> (66.9109, -57.5538)
  line L30 (66.9109, -57.5538) -> (67.113, -57.4925)
  line L31 (67.113, -57.4925) -> (67.3133, -57.4259)
  line L32 (67.3133, -57.4259) -> (67.5118, -57.354)
  line L33 (67.5118, -57.354) -> (67.6696, -57.7725)
  line L34 (67.6696, -57.7725) -> (67.7008, -57.8376)
  line L35 (67.7008, -57.8376) -> (67.737, -57.9008)
  line L36 (67.737, -57.9008) -> (67.7764, -57.9627)
  line L37 (67.7764, -57.9627) -> (67.8186, -58.0235)
  line L38 (67.8186, -58.0235) -> (67.8632, -58.0834)
  line L39 (67.8632, -58.0834) -> (67.9099, -58.1424)
  line L40 (67.9099, -58.1424) -> (67.9586, -58.2006)
  line L41 (67.9586, -58.2006) -> (68.0092, -58.2579)
  line L42 (68.0092, -58.2579) -> (68.0616, -58.3145)
  line L43 (68.0616, -58.3145) -> (68.1157, -58.3702)
  line L44 (68.1157, -58.3702) -> (68.1715, -58.4252)
  line L45 (68.1715, -58.4252) -> (68.2288, -58.4794)
  line L46 (68.2288, -58.4794) -> (68.3583, -58.4251)
  line L47 (68.3583, -58.4251) -> (68.487, -58.3688)
  line L48 (68.487, -58.3688) -> (68.6148, -58.3106)
  line L49 (68.6148, -58.3106) -> (68.6139, -58.2316)
  line L50 (68.6139, -58.2316) -> (68.6113, -58.1534)
  line L51 (68.6113, -58.1534) -> (68.6071, -58.0758)
  line L52 (68.6071, -58.0758) -> (68.6011, -57.9989)
  line L53 (68.6011, -57.9989) -> (68.5933, -57.9228)
  line L54 (68.5933, -57.9228) -> (68.5837, -57.8476)
  line L55 (68.5837, -57.8476) -> (68.572, -57.7732)
  line L56 (68.572, -57.7732) -> (68.5583, -57.6999)
  line L57 (68.5583, -57.6999) -> (68.5422, -57.6276)
  line L58 (68.5422, -57.6276) -> (68.5235, -57.5566)
  line L59 (68.5235, -57.5566) -> (68.5016, -57.4872)
  line L60 (68.5016, -57.4872) -> (68.475, -57.4201)
  line L61 (68.475, -57.4201) -> (68.2747, -57.0202)
  line L62 (68.2747, -57.0202) -> (68.4622, -56.9232)
  line L63 (68.4622, -56.9232) -> (68.6471, -56.8212)
  line L64 (68.6471, -56.8212) -> (68.8292, -56.7144)
  line L65 (68.8292, -56.7144) -> (69.0084, -56.6028)
  line L66 (69.0084, -56.6028) -> (69.2497, -56.9794)
  line L67 (69.2497, -56.9794) -> (69.2938, -57.0365)
  line L68 (69.2938, -57.0365) -> (69.3423, -57.0908)
  line L69 (69.3423, -57.0908) -> (69.3938, -57.1432)
  line L70 (69.3938, -57.1432) -> (69.4477, -57.1939)
  line L71 (69.4477, -57.1939) -> (69.5037, -57.2432)
  line L72 (69.5037, -57.2432) -> (69.5617, -57.2912)
  line L73 (69.5617, -57.2912) -> (69.6215, -57.338)
  line L74 (69.6215, -57.338) -> (69.6829, -57.3836)
  line L75 (69.6829, -57.3836) -> (69.7459, -57.428)
  line L76 (69.7459, -57.428) -> (69.8104, -57.4713)
  line L77 (69.8104, -57.4713) -> (69.8764, -57.5135)
  line L78 (69.8764, -57.5135) -> (69.9438, -57.5546)
  line L79 (69.9438, -57.5546) -> (70.0591, -57.4745)
  line L80 (70.0591, -57.4745) -> (70.1733, -57.3927)
  line L81 (70.1733, -57.3927) -> (70.2861, -57.3092)
  line L82 (70.2861, -57.3092) -> (70.2688, -57.2322)
  line L83 (70.2688, -57.2322) -> (70.2501, -57.1561)
  line L84 (70.2501, -57.1561) -> (70.2298, -57.0811)
  line L85 (70.2298, -57.0811) -> (70.208, -57.0072)
  line L86 (70.208, -57.0072) -> (70.1845, -56.9344)
  line L87 (70.1845, -56.9344) -> (70.1595, -56.8628)
  line L88 (70.1595, -56.8628) -> (70.1326, -56.7925)
  line L89 (70.1326, -56.7925) -> (70.1039, -56.7236)
  line L90 (70.1039, -56.7236) -> (70.0732, -56.6562)
  line L91 (70.0732, -56.6562) -> (70.0401, -56.5907)
  line L92 (70.0401, -56.5907) -> (70.0043, -56.5273)
  line L93 (70.0043, -56.5273) -> (69.9643, -56.4672)
  line L94 (69.9643, -56.4672) -> (69.6852, -56.1177)
  line L95 (69.6852, -56.1177) -> (69.8485, -55.9838)
  line L96 (69.8485, -55.9838) -> (70.0081, -55.8456)
  line L97 (70.0081, -55.8456) -> (70.164, -55.7033)
  line L98 (70.164, -55.7033) -> (70.3162, -55.5569)
  line L99 (70.3162, -55.5569) -> (70.6305, -55.8751)
  line L100 (70.6305, -55.8751) -> (70.6855, -55.9218)
  line L101 (70.6855, -55.9218) -> (70.7442, -55.9648)
  line L102 (70.7442, -55.9648) -> (70.8054, -56.0053)
  line L103 (70.8054, -56.0053) -> (70.8687, -56.0437)
  line L104 (70.8687, -56.0437) -> (70.9338, -56.0803)
  line L105 (70.9338, -56.0803) -> (71.0005, -56.1152)
  line L106 (71.0005, -56.1152) -> (71.0686, -56.1485)
  line L107 (71.0686, -56.1485) -> (71.1382, -56.1803)
  line L108 (71.1382, -56.1803) -> (71.209, -56.2107)
  line L109 (71.209, -56.2107) -> (71.2812, -56.2396)
  line L110 (71.2812, -56.2396) -> (71.3545, -56.2672)
  line L111 (71.3545, -56.2672) -> (71.4289, -56.2934)
  line L112 (71.4289, -56.2934) -> (71.5251, -56.1911)
  line L113 (71.5251, -56.1911) -> (71.6197, -56.0873)
  line L114 (71.6197, -56.0873) -> (71.7128, -55.9821)
  line L115 (71.7128, -55.9821) -> (71.6799, -55.9104)
  line L116 (71.6799, -55.9104) -> (71.6457, -55.8399)
  line L117 (71.6457, -55.8399) -> (71.6103, -55.7708)
  line L118 (71.6103, -55.7708) -> (71.5735, -55.703)
  line L119 (71.5735, -55.703) -> (71.5355, -55.6367)
  line L120 (71.5355, -55.6367) -> (71.4961, -55.5718)
  line L121 (71.4961, -55.5718) -> (71.4552, -55.5086)
  line L122 (71.4552, -55.5086) -> (71.4128, -55.4472)
  line L123 (71.4128, -55.4472) -> (71.3687, -55.3877)
  line L124 (71.3687, -55.3877) -> (71.3227, -55.3305)
  line L125 (71.3227, -55.3305) -> (71.2745, -55.2759)
  line L126 (71.2745, -55.2759) -> (71.2229, -55.2255)
  line L127 (71.2229, -55.2255) -> (70.8773, -54.9417)
  line L128 (70.8773, -54.9417) -> (71.0091, -54.7767)
  line L129 (71.0091, -54.7767) -> (71.1365, -54.6084)
  line L130 (71.1365, -54.6084) -> (71.2595, -54.4368)
  line L131 (71.2595, -54.4368) -> (71.3778, -54.2619)
  line L132 (71.3778, -54.2619) -> (71.7514, -54.5078)
  line L133 (71.7514, -54.5078) -> (71.8149, -54.5421)
  line L134 (71.8149, -54.5421) -> (71.8813, -54.5719)
  line L135 (71.8813, -54.5719) -> (71.9497, -54.5988)
  line L136 (71.9497, -54.5988) -> (72.0195, -54.6232)
  line L137 (72.0195, -54.6232) -> (72.0908, -54.6455)
  line L138 (72.0908, -54.6455) -> (72.1633, -54.6658)
  line L139 (72.1633, -54.6658) -> (72.2369, -54.6842)
  line L140 (72.2369, -54.6842) -> (72.3115, -54.7008)
  line L141 (72.3115, -54.7008) -> (72.3871, -54.7158)
  line L142 (72.3871, -54.7158) -> (72.4637, -54.7291)
  line L143 (72.4637, -54.7291) -> (72.5411, -54.7408)
  line L144 (72.5411, -54.7408) -> (72.6194, -54.751)
  line L145 (72.6194, -54.751) -> (72.6922, -54.6309)
  line L146 (72.6922, -54.6309) -> (72.7632, -54.5097)
  line L147 (72.7632, -54.5097) -> (72.8324, -54.3875)
  line L148 (72.8324, -54.3875) -> (72.7852, -54.3242)
  line L149 (72.7852, -54.3242) -> (72.7372, -54.2624)
  line L150 (72.7372, -54.2624) -> (72.6881, -54.2021)
  line L151 (72.6881, -54.2021) -> (72.6381, -54.1434)
  line L152 (72.6381, -54.1434) -> (72.5871, -54.0864)
  line L153 (72.5871, -54.0864) -> (72.5351, -54.0312)
  line L154 (72.5351, -54.0312) -> (72.4819, -53.9779)
  line L155 (72.4819, -53.9779) -> (72.4277, -53.9266)
  line L156 (72.4277, -53.9266) -> (72.3722, -53.8776)
  line L157 (72.3722, -53.8776) -> (72.3154, -53.8312)
  line L158 (72.3154, -53.8312) -> (72.2568, -53.7879)
  line L159 (72.2568, -53.7879) -> (72.1959, -53.7492)
  line L160 (72.1959, -53.7492) -> (71.7988, -53.5435)
  line L161 (71.7988, -53.5435) -> (71.8934, -53.3547)
  line L162 (71.8934, -53.3547) -> (71.9831, -53.1636)
  line L163 (71.9831, -53.1636) -> (72.0676, -52.9701)
  line L164 (72.0676, -52.9701) -> (72.1471, -52.7745)
  line L165 (72.1471, -52.7745) -> (72.5636, -52.9373)
  line L166 (72.5636, -52.9373) -> (72.6329, -52.9577)
  line L167 (72.6329, -52.9577) -> (72.704, -52.973)
  line L168 (72.704, -52.973) -> (72.7764, -52.9852)
  line L169 (72.7764, -52.9852) -> (72.8499, -52.9945)
  line L170 (72.8499, -52.9945) -> (72.9242, -53.0015)
  line L171 (72.9242, -53.0015) -> (72.9993, -53.0063)
  line L172 (72.9993, -53.0063) -> (73.0751, -53.009)
  line L173 (73.0751, -53.009) -> (73.1516, -53.0097)
  line L174 (73.1516, -53.0097) -> (73.2287, -53.0086)
  line L175 (73.2287, -53.0086) -> (73.3063, -53.0057)
  line L176 (73.3063, -53.0057) -> (73.3845, -53.0011)
  line L177 (73.3845, -53.0011) -> (73.4632, -52.9947)
  line L178 (73.4632, -52.9947) -> (73.5094, -52.8621)
  line L179 (73.5094, -52.8621) -> (73.5537, -52.7289)
  line L180 (73.5537, -52.7289) -> (73.5959, -52.5949)
  line L181 (73.5959, -52.5949) -> (73.5367, -52.5428)
  line L182 (73.5367, -52.5428) -> (73.4768, -52.4923)
  line L183 (73.4768, -52.4923) -> (73.4163, -52.4436)
  line L184 (73.4163, -52.4436) -> (73.3552, -52.3966)
  line L185 (73.3552, -52.3966) -> (73.2934, -52.3514)
  line L186 (73.2934, -52.3514) -> (73.231, -52.3083)
  line L187 (73.231, -52.3083) -> (73.168, -52.2672)
  line L188 (73.168, -52.2672) -> (73.1043, -52.2283)
  line L189 (73.1043, -52.2283) -> (73.0398, -52.1919)
  line L190 (73.0398, -52.1919) -> (72.9745, -52.1583)
  line L191 (72.9745, -52.1583) -> (72.9083, -52.128)
  line L192 (72.9083, -52.128) -> (72.8407, -52.1029)
  line L193 (72.8407, -52.1029) -> (72.4095, -51.9842)
  line L194 (72.4095, -51.9842) -> (72.4628, -51.78)
  line L195 (72.4628, -51.78) -> (72.5107, -51.5744)
  line L196 (72.5107, -51.5744) -> (72.5532, -51.3675)
  line L197 (72.5532, -51.3675) -> (72.5902, -51.1597)
  line L198 (72.5902, -51.1597) -> (73.0315, -51.2323)
  line L199 (73.0315, -51.2323) -> (73.1035, -51.2378)
  line L200 (73.1035, -51.2378) -> (73.1763, -51.2381)
  line L201 (73.1763, -51.2381) -> (73.2497, -51.2349)
  line L202 (73.2497, -51.2349) -> (73.3234, -51.2288)
  line L203 (73.3234, -51.2288) -> (73.3976, -51.2201)
  line L204 (73.3976, -51.2201) -> (73.472, -51.2092)
  line L205 (73.472, -51.2092) -> (73.5468, -51.196)
  line L206 (73.5468, -51.196) -> (73.6217, -51.1809)
  line L207 (73.6217, -51.1809) -> (73.6969, -51.1638)
  line L208 (73.6969, -51.1638) -> (73.7722, -51.1448)
  line L209 (73.7722, -51.1448) -> (73.8477, -51.124)
  line L210 (73.8477, -51.124) -> (73.9234, -51.1015)
  line L211 (73.9234, -51.1015) -> (73.9411, -50.9621)
  line L212 (73.9411, -50.9621) -> (73.9566, -50.8226)
  line L213 (73.9566, -50.8226) -> (73.9701, -50.6828)
  line L214 (73.9701, -50.6828) -> (73.9013, -50.6441)
  line L215 (73.9013, -50.6441) -> (73.8322, -50.6072)
  line L216 (73.8322, -50.6072) -> (73.7629, -50.5721)
  line L217 (73.7629, -50.5721) -> (73.6934, -50.5388)
  line L218 (73.6934, -50.5388) -> (73.6236, -50.5075)
  line L219 (73.6236, -50.5075) -> (73.5536, -50.4782)
  line L220 (73.5536, -50.4782) -> (73.4834, -50.4511)
  line L221 (73.4834, -50.4511) -> (73.413, -50.4264)
  line L222 (73.413, -50.4264) -> (73.3424, -50.4042)
  line L223 (73.3424, -50.4042) -> (73.2715, -50.3849)
  line L224 (73.2715, -50.3849) -> (73.2004, -50.3691)
  line L225 (73.2004, -50.3691) -> (73.129, -50.3585)
  line L226 (73.129, -50.3585) -> (72.6826, -50.3321)
  line L227 (72.6826, -50.3321) -> (72.6923, -50.1212)
  line L228 (72.6923, -50.1212) -> (72.6964, -49.9101)
  line L229 (72.6964, -49.9101) -> (72.695, -49.699)
  line L230 (72.695, -49.699) -> (72.688, -49.488)
  line L231 (72.688, -49.488) -> (73.1348, -49.4673)
  line L232 (73.1348, -49.4673) -> (73.2063, -49.4577)
  line L233 (73.2063, -49.4577) -> (73.2775, -49.4428)
  line L234 (73.2775, -49.4428) -> (73.3486, -49.4244)
  line L235 (73.3486, -49.4244) -> (73.4195, -49.4031)
  line L236 (73.4195, -49.4031) -> (73.4903, -49.3793)
  line L237 (73.4903, -49.3793) -> (73.5608, -49.3531)
  line L238 (73.5608, -49.3531) -> (73.6312, -49.3247)
  line L239 (73.6312, -49.3247) -> (73.7013, -49.2943)
  line L240 (73.7013, -49.2943) -> (73.7713, -49.2619)
  line L241 (73.7713, -49.2619) -> (73.8411, -49.2277)
  line L242 (73.8411, -49.2277) -> (73.9106, -49.1916)
  line L243 (73.9106, -49.1916) -> (73.9799, -49.1539)
  line L244 (73.9799, -49.1539) -> (73.9682, -49.0139)
  line L245 (73.9682, -49.0139) -> (73.9544, -48.8742)
  line L246 (73.9544, -48.8742) -> (73.9385, -48.7346)
  line L247 (73.9385, -48.7346) -> (73.8632, -48.7111)
  line L248 (73.8632, -48.7111) -> (73.788, -48.6894)
  line L249 (73.788, -48.6894) -> (73.7129, -48.6694)
  line L250 (73.7129, -48.6694) -> (73.6379, -48.6513)
  line L251 (73.6379, -48.6513) -> (73.5632, -48.6352)
  line L252 (73.5632, -48.6352) -> (73.4886, -48.6212)
  line L253 (73.4886, -48.6212) -> (73.4143, -48.6092)
  line L254 (73.4143, -48.6092) -> (73.3403, -48.5997)
  line L255 (73.3403, -48.5997) -> (73.2666, -48.5926)
  line L256 (73.2666, -48.5926) -> (73.1933, -48.5885)
  line L257 (73.1933, -48.5885) -> (73.1205, -48.5878)
  line L258 (73.1205, -48.5878) -> (73.0485, -48.5923)
  line L259 (73.0485, -48.5923) -> (72.6063, -48.6593)
  line L260 (72.6063, -48.6593) -> (72.5719, -48.451)
  line L261 (72.5719, -48.451) -> (72.5321, -48.2437)
  line L262 (72.5321, -48.2437) -> (72.4868, -48.0375)
  line L263 (72.4868, -48.0375) -> (72.436, -47.8325)
  line L264 (72.436, -47.8325) -> (72.8687, -47.7194)
  line L265 (72.8687, -47.7194) -> (72.9367, -47.6951)
  line L266 (72.9367, -47.6951) -> (73.0033, -47.6658)
  line L267 (73.0033, -47.6658) -> (73.069, -47.633)
  line L268 (73.069, -47.633) -> (73.1339, -47.5974)
  line L269 (73.1339, -47.5974) -> (73.1982, -47.5594)
  line L270 (73.1982, -47.5594) -> (73.2617, -47.5191)
  line L271 (73.2617, -47.5191) -> (73.3247, -47.4767)
  line L272 (73.3247, -47.4767) -> (73.387, -47.4323)
  line L273 (73.387, -47.4323) -> (73.4487, -47.3861)
  line L274 (73.4487, -47.3861) -> (73.5098, -47.3381)
  line L275 (73.5098, -47.3381) -> (73.5703, -47.2884)
  line L276 (73.5703, -47.2884) -> (73.6302, -47.2371)
  line L277 (73.6302, -47.2371) -> (73.5897, -47.1026)
  line L278 (73.5897, -47.1026) -> (73.5472, -46.9688)
  line L279 (73.5472, -46.9688) -> (73.5026, -46.8356)
  line L280 (73.5026, -46.8356) -> (73.424, -46.8283)
  line L281 (73.424, -46.8283) -> (73.3459, -46.8226)
  line L282 (73.3459, -46.8226) -> (73.2683, -46.8187)
  line L283 (73.2683, -46.8187) -> (73.1913, -46.8166)
  line L284 (73.1913, -46.8166) -> (73.1148, -46.8164)
  line L285 (73.1148, -46.8164) -> (73.0389, -46.8182)
  line L286 (73.0389, -46.8182) -> (72.9638, -46.822)
  line L287 (72.9638, -46.822) -> (72.8894, -46.828)
  line L288 (72.8894, -46.828) -> (72.8158, -46.8364)
  line L289 (72.8158, -46.8364) -> (72.7433, -46.8476)
  line L290 (72.7433, -46.8476) -> (72.6719, -46.8621)
  line L291 (72.6719, -46.8621) -> (72.6024, -46.8815)
  line L292 (72.6024, -46.8815) -> (72.1838, -47.0389)
  line L293 (72.1838, -47.0389) -> (72.1069, -46.8423)
  line L294 (72.1069, -46.8423) -> (72.0248, -46.6478)
  line L295 (72.0248, -46.6478) -> (71.9376, -46.4555)
  line L296 (71.9376, -46.4555) -> (71.8454, -46.2656)
  line L297 (71.8454, -46.2656) -> (72.2451, -46.065)
  line L298 (72.2451, -46.065) -> (72.3066, -46.0271)
  line L299 (72.3066, -46.0271) -> (72.3656, -45.9845)
  line L300 (72.3656, -45.9845) -> (72.4231, -45.9388)
  line L301 (72.4231, -45.9388) -> (72.4792, -45.8905)
  line L302 (72.4792, -45.8905) -> (72.5341, -45.8399)
  line L303 (72.5341, -45.8399) -> (72.5879, -45.7873)
  line L304 (72.5879, -45.7873) -> (72.6406, -45.7328)
  line L305 (72.6406, -45.7328) -> (72.6923, -45.6765)
  line L306 (72.6923, -45.6765) -> (72.7431, -45.6184)
  line L307 (72.7431, -45.6184) -> (72.7929, -45.5588)
  line L308 (72.7929, -45.5588) -> (72.8418, -45.4976)
  line L309 (72.8418, -45.4976) -> (72.8897, -45.4349)
  line L310 (72.8897, -45.4349) -> (72.8221, -45.3118)
  line L311 (72.8221, -45.3118) -> (72.7527, -45.1897)
  line L312 (72.7527, -45.1897) -> (72.6814, -45.0687)
  line L313 (72.6814, -45.0687) -> (72.603, -45.0779)
  line L314 (72.603, -45.0779) -> (72.5254, -45.0886)
  line L315 (72.5254, -45.0886) -> (72.4487, -45.1009)
  line L316 (72.4487, -45.1009) -> (72.3729, -45.1149)
  line L317 (72.3729, -45.1149) -> (72.2981, -45.1306)
  line L318 (72.2981, -45.1306) -> (72.2242, -45.148)
  line L319 (72.2242, -45.148) -> (72.1515, -45.1674)
  line L320 (72.1515, -45.1674) -> (72.08, -45.1887)
  line L321 (72.08, -45.1887) -> (72.0098, -45.2123)
  line L322 (72.0098, -45.2123) -> (71.9411, -45.2383)
  line L323 (71.9411, -45.2383) -> (71.8743, -45.2673)
  line L324 (71.8743, -45.2673) -> (71.8104, -45.3008)
  line L325 (71.8104, -45.3008) -> (71.4337, -45.5418)
  line L326 (71.4337, -45.5418) -> (71.3176, -45.3655)
  line L327 (71.3176, -45.3655) -> (71.1968, -45.1923)
  line L328 (71.1968, -45.1923) -> (71.0716, -45.0223)
  line L329 (71.0716, -45.0223) -> (70.9419, -44.8557)
  line L330 (70.9419, -44.8557) -> (71.2912, -44.5764)
  line L331 (71.2912, -44.5764) -> (71.3434, -44.5266)
  line L332 (71.3434, -44.5266) -> (71.3923, -44.4726)
  line L333 (71.3923, -44.4726) -> (71.439, -44.416)
  line L334 (71.439, -44.416) -> (71.4838, -44.3571)
  line L335 (71.4838, -44.3571) -> (71.527, -44.2962)
  line L336 (71.527, -44.2962) -> (71.5687, -44.2335)
  line L337 (71.5687, -44.2335) -> (71.6089, -44.1692)
  line L338 (71.6089, -44.1692) -> (71.6478, -44.1034)
  line L339 (71.6478, -44.1034) -> (71.6854, -44.036)
  line L340 (71.6854, -44.036) -> (71.7217, -43.9674)
  line L341 (71.7217, -43.9674) -> (71.7568, -43.8973)
  line L342 (71.7568, -43.8973) -> (71.7907, -43.826)
  line L343 (71.7907, -43.826) -> (71.6989, -43.7197)
  line L344 (71.6989, -43.7197) -> (71.6057, -43.6147)
  line L345 (71.6057, -43.6147) -> (71.5108, -43.5112)
  line L346 (71.5108, -43.5112) -> (71.436, -43.5364)
  line L347 (71.436, -43.5364) -> (71.3624, -43.5631)
  line L348 (71.3624, -43.5631) -> (71.2899, -43.5911)
  line L349 (71.2899, -43.5911) -> (71.2186, -43.6205)
  line L350 (71.2186, -43.6205) -> (71.1487, -43.6514)
  line L351 (71.1487, -43.6514) -> (71.0801, -43.6838)
  line L352 (71.0801, -43.6838) -> (71.013, -43.7179)
  line L353 (71.013, -43.7179) -> (70.9474, -43.7536)
  line L354 (70.9474, -43.7536) -> (70.8837, -43.7912)
  line L355 (70.8837, -43.7912) -> (70.8219, -43.831)
  line L356 (70.8219, -43.831) -> (70.7626, -43.8732)
  line L357 (70.7626, -43.8732) -> (70.7071, -43.9192)
  line L358 (70.7071, -43.9192) -> (70.3887, -44.2333)
  line L359 (70.3887, -44.2333) -> (70.2384, -44.085)
  line L360 (70.2384, -44.085) -> (70.0843, -43.9407)
  line L361 (70.0843, -43.9407) -> (69.9265, -43.8005)
  line L362 (69.9265, -43.8005) -> (69.765, -43.6645)
  line L363 (69.765, -43.6645) -> (70.0486, -43.3186)
  line L364 (70.0486, -43.3186) -> (70.0893, -43.2591)
  line L365 (70.0893, -43.2591) -> (70.1259, -43.1961)
  line L366 (70.1259, -43.1961) -> (70.1598, -43.131)
  line L367 (70.1598, -43.131) -> (70.1914, -43.0641)
  line L368 (70.1914, -43.0641) -> (70.221, -42.9955)
  line L369 (70.221, -42.9955) -> (70.2487, -42.9256)
  line L370 (70.2487, -42.9256) -> (70.2747, -42.8543)
  line L371 (70.2747, -42.8543) -> (70.2991, -42.7818)
  line L372 (70.2991, -42.7818) -> (70.3219, -42.7081)
  line L373 (70.3219, -42.7081) -> (70.3431, -42.6334)